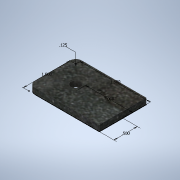
# Autodesk Inventor part: 1
Saved by Autodesk Inventor 2021 (Build 250183000, 183)
## iProperties
Created: 2020-11-06
Part Number: 1
Material: Steel
Document SubType Name: Modeling
Designer: mackeycj
Density: 7.85 g/cm^3
Appearance: Plate
Mass: 11.7508 g
Surface Area: 21.0863 cm^2
Volume: 1.49692 cm^3
Description: floor mount tab
Author: mackeycj
Title: Floor Tabs
Autodesk Inventor part; units mm, degrees
ref_plane "YZ Plane" through (0, 0, 0) normal (1, 0, 0) x (0, 1, 0)
ref_plane "XZ Plane" through (0, 0, 0) normal (0, 1, 0) x (-1, 0, 0)
ref_plane "XY Plane" through (0, 0, 0) normal (0, 0, 1) x (1, 0, 0)
sketch "Sketch1" plane through (0, 0, 0) normal (0, 1, 0) x (-1, 0, 0)
  line L0 (0, 0) -> (34.925, 0)
  line L1 (38.1, -3.175) -> (38.1, -22.225)
  line L2 (34.925, -25.4) -> (0, -25.4)
  line L3 (0, -25.4) -> (0, 0)
  line L4 (0, 0) -> (0, -12.7)
  line L5 (0, -12.7) -> (25.4, -12.7)
  arc A0 (34.925, -25.4) -> (38.1, -22.225) centre (34.925, -22.225) ccw
  arc A1 (38.1, -3.175) -> (34.925, 0) centre (34.925, -3.175) ccw
  point P0 (38.1, -25.4)
  point P1 (38.1, 0)
  dimension "d0" = 38.1
  dimension "d1" = 25.4
  dimension "d2" = 12.7
  dimension "d3" = 25.4
  dimension "d7" = 3.175
  constraints: 12 end point, 4 point on circle, 4 point on line, 4 tangent, 2 centre point, 2 parallel, 2 perpendicular, 1 equal radius, 1 horizontal, 1 midpoint
  measures "d0" distance of point (38.1, -25.4) L2.end
  measures "d1" distance of point (38.1, 0) point (38.1, -25.4)
  measures "d2" distance of L0.start L4.end
  measures "d3" distance of L4.end L5.end
  measures "d7" radius of A0
extrude "Extrusion1" add sketch "Sketch1" along normal blind 3.175
hole "Hole1" at (-25.4, 0, -12.7) direction (0, 1, 0) diameter 5.1054 end through all clearance for "Flat Head Machine Screw (82)" size "#10" standard "Ansi Unified Screw Threads"
body "Solid1"
